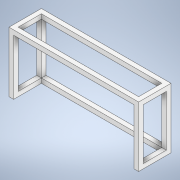
# Autodesk Inventor part: Goal
Saved by Autodesk Inventor 2022 (Build 260153000, 153)
## iProperties
Created: 2022-10-30
Part Number: Goal
Material: 一般
Document SubType Name: Modeling
Designer: Masato Kubotera
Density: 1 g/cm^3
Appearance: 既定
Author: Masato Kubotera
Autodesk Inventor part; units mm, degrees
ref_plane "YZ Plane" through (0, 0, 0) normal (1, 0, 0) x (0, 1, 0)
ref_plane "XZ Plane" through (0, 0, 0) normal (0, 1, 0) x (-1, 0, 0)
ref_plane "XY Plane" through (0, 0, 0) normal (0, 0, 1) x (1, 0, 0)
sketch "スケッチ1" plane through (0, 0, 0) normal (0, 0, 1) x (1, 0, 0)
  line L0 (-300, 1350) -> (300, 1350) construction
  line L1 (300, 1350) -> (300, -1350) construction
  line L2 (300, -1350) -> (-300, -1350) construction
  line L3 (-300, -1350) -> (-300, 1350) construction
  line L4 (-300, 1350) -> (300, -1350) construction
  line L5 (300, 1350) -> (-300, -1350) construction
  line L6 (350, 1400) -> (-350, 1400)
  line L7 (-350, 1400) -> (-350, 1300)
  line L8 (-350, 1300) -> (-250, 1300)
  line L9 (250, 1300) -> (250, -1300)
  line L10 (250, -1300) -> (-250, -1300)
  line L11 (-350, -1300) -> (-350, -1400)
  line L12 (-350, -1400) -> (350, -1400)
  line L13 (350, -1400) -> (350, 1400)
  line L14 (350, 0) -> (-300, 0) construction
  line L15 (-350, 1300) -> (-350, -1300)
  line L16 (-250, -1400) -> (-250, -1300)
  line L17 (250, 1300) -> (250, 1400)
  line L18 (250, -1300) -> (250, -1400)
  line L19 (250, -1300) -> (350, -1300)
  line L20 (250, 1300) -> (350, 1300)
  line L21 (-250, 1300) -> (-250, 1350)
  line L22 (-250, -1300) -> (-250, 1300)
  line L23 (-250, 1350) -> (-250, 1400)
  line L24 (-250, 1300) -> (250, 1300)
  line L25 (-250, -1300) -> (-350, -1300)
  point P0 (0, 0)
  point P1 (0, 0)
  point P2 (0, 0)
  dimension "d2" = 100
  dimension "d3" = 100
  dimension "d5" = 100
  dimension "d12" = 600
  dimension "d13" = 2600
  constraints: 52 end point, 17 perpendicular, 8 point on line, 5 midpoint, 4 parallel, 2 horizontal, 1 coincident, 1 collinear, 6 other
  measures "d2" distance between parallel lines of L6 L8
  measures "d3" distance between parallel lines of L13 L9
  measures "d5" distance between parallel lines of L16 L15
  measures "d12" distance between parallel lines of L15 L9
  measures "d13" distance between parallel lines of L25 L8
extrude "押し出し1" add sketch "スケッチ1" along normal blind 1300 contours L13 L20 L17 L6 | L17 L24 L21 L23 L6 | L13 L19 L9 L20 | L23 L21 L8 L7 L6 | L13 L12 L18 L19 | L18 L12 L16 L10 | L22 L25 L15 L8 | L16 L12 L11 L25
extrude "押し出し2" cut sketch "スケッチ1" along normal blind 1200 contours L17 L24 L21 L23 L6 | L13 L19 L9 L20 | L9 L10 L22 L24 | L18 L12 L16 L10 | L22 L25 L15 L8
extrude "押し出し3" add sketch "スケッチ1" along normal blind 100 contours L17 L24 L21 L23 L6 | L13 L19 L9 L20 | L18 L12 L16 L10
equation "\"d3\" = d2"
equation "\"d5\" = d2"
